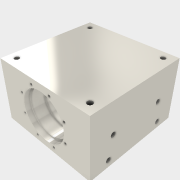
# Autodesk Inventor part: PWTR-0045
Saved by Autodesk Inventor 2021.1 (Build 251245000, 245)
## iProperties
Created: 2020-08-27
Part Number: PWTR-0045
Material: Aluminum 6061
Document SubType Name: Modeling
Designer: alid
Density: 2.7 g/cm^3
Appearance: Titanium - Polished
Description: Transfer Box Casing
Mass: 2475.75 g
Surface Area: 1069.23 cm^2
Volume: 916.945 cm^3
Author: alid
Revision Number: A
Autodesk Inventor part; units mm, degrees
ref_plane "YZ Plane" through (0, 0, 0) normal (1, 0, 0) x (0, 1, 0)
ref_plane "XZ Plane" through (0, 0, 0) normal (0, 1, 0) x (-1, 0, 0)
ref_plane "XY Plane" through (0, 0, 0) normal (0, 0, 1) x (1, 0, 0)
sketch "Sketch1" plane through (0, 0, 0) normal (0, 0, 1) x (1, 0, 0)
  line L0 (-65, -65) -> (65, -65)
  line L1 (65, -65) -> (65, 65)
  line L2 (65, 65) -> (-65, 65)
  line L3 (-65, 65) -> (-65, -65)
  line L4 (-65, -65) -> (65, 65) construction
  line L5 (65, -65) -> (-65, 65) construction
  circle A0 centre (0, 0) radius 50 construction
  circle A1 centre (0, 0) radius 75 construction
  point P0 (35.3553, 35.3553)
  point P1 (53.033, 53.033)
  dimension "d4" = 100
  dimension "d22" = 150
  dimension "d0" = 130
  dimension "d1" = 130
  constraints: 12 end point, 2 coincident, 2 midpoint, 2 parallel, 2 point on line, 1 horizontal, 1 perpendicular, 6 other
  measures "d0" distance of L2.end L1.end
  measures "d1" distance of L1.end L0.end
extrude "Extrusion1" add sketch "Sketch1" along normal blind 80
hole "Hole1" at (35.3553, 35.3553, 0) direction (0, 0, 1) diameter 6.647 depth 22.2 tip angle 118 thread size "M8x1.25" class "6H" standard "ISO Metric profile"
hole "Hole2" at (0, 0, 0) direction (0, 0, 1) diameter 75 depth 70
pattern_circular "Circular Pattern1" count 4 over 360 about axis through (0, 0, -10) along (0, 0, 1) of "Hole1"
hole "Hole3" at (53.033, 53.033, 0) direction (0, 0, 1) diameter 6.647 end through all thread size "M8x1.25" class "6H" standard "ISO Metric profile"
pattern_circular "Circular Pattern2" count 4 over 360 about axis through (0, 0, -10) along (0, 0, 1) of "Hole3"
sketch "Sketch2" plane through (0, 0, 0) normal (0, 1, 0) x (-1, 0, 0)
  line L0 (0, 40) -> (65, 40)
  line L1 (0, 66) -> (0, 40)
  line L2 (65, 47.2135) -> (65, 40)
  line L3 (65, 0) -> (65, 80) projected
  line L4 (0, 66) -> (41, 66)
  line L5 (41, 66) -> (41, 69)
  line L6 (41, 69) -> (65, 69)
  line L7 (0, 61) -> (-49.5, 61)
  line L8 (-49.5, 61) -> (-52.5, 58)
  line L9 (-52.5, 58) -> (-52.5, 50)
  line L10 (-52.5, 50) -> (-65, 50)
  line L11 (-65, 50) -> (-65, 40)
  line L12 (-65, 40) -> (0, 40)
  line L13 (58, 69) -> (58, 71)
  line L14 (58, 71) -> (65, 71)
  line L15 (65, 69) -> (65, 71)
  point P0 (0, 0)
  dimension "d36" = 40
  dimension "d42" = 41
  dimension "d43" = 26
  dimension "d44" = 29
  dimension "d45" = 42
  dimension "d46" = 135
  dimension "d47" = 3
  dimension "d48" = 20
  dimension "d50" = 65
  dimension "d51" = 49.5
  dimension "d59" = 7
  dimension "d60" = 31
  constraints: 30 end point, 8 perpendicular, 5 point on line, 2 horizontal, 2 vertical, 2 vertical alignment, 1 midpoint, 1 parallel
  measures "d36" distance from line of L3.start L0
  measures "d42" distance between parallel lines of L5 L1
  measures "d43" distance from line of L0.start L4
  measures "d44" distance from line of L0.start L6
  measures "d45" diameter of L7 L12
  measures "d46" angle of L9 L8
  measures "d47" horizontal distance of L7.end L8.end
  measures "d48" diameter of L10 L12
  measures "d50" distance from line of L0.start L11
  measures "d51" distance from line of L7.end L1
  measures "d59" distance of L13.end L14.end
  measures "d60" distance from line of L0.start L14
revolve "Revolution1" cut sketch "Sketch2" angle 360 about axis through (0, 0, 40) along (-1, 0, 0)
sketch "Sketch3" plane through (65, -65, 0) normal (1, 0, 0) x (0, 0, -1)
  circle A0 centre (-40, 65) radius 10 projected
  point P0 (0, 65)
  constraints: 1 coincident
hole "Hole4" at (65, 0, 40) direction (-1, 0, 0) diameter 30 depth 7
sketch "Sketch4" plane through (-65, -65, 0) normal (-1, 0, 0) x (0, 0, 1)
  circle A0 centre (40, 65) radius 31 projected
  circle A1 centre (40, 65) radius 40 construction
  circle A2 centre (40, 65) radius 35 construction
  line L0 (40, 65) -> (75, 65) construction
  line L1 (40, 65) -> (72.3358, 51.6061) construction
  point P0 (0, 65)
  dimension "d61" = 80
  dimension "d62" = 70
  dimension "d63" = 22.5
  constraints: 4 end point, 2 centre point, 2 coincident, 2 point on circle, 1 horizontal
  measures "d61" diameter of A1
  measures "d62" diameter of A2
  measures "d63" angle of L1 L0
hole "Hole5" at (-65, -13.3939, 72.3358) direction (1, 0, 0) diameter 3.242 depth 11.8 thread size "M4x0.7" class "6H" standard "ISO Metric profile"
pattern_circular "Circular Pattern3" count 8 over 360 about axis through (-61.5, 0, 40) along (1, 0, 0) of "Hole5"
sketch "Sketch5" plane through (-65, -65, 0) normal (0, -1, 0) x (1, 0, 0)
  line L0 (25, 0) -> (105, 0)
  line L1 (100, 50) -> (30, 50)
  line L2 (109.8639, 41.644) -> (114.8639, 11.644)
  circle A0 centre (30, 40) radius 10
  circle A1 centre (25, 10) radius 10
  circle A2 centre (100, 40) radius 10
  circle A3 centre (105, 10) radius 10
  line L3 (20.1361, 41.644) -> (15.1361, 11.644)
  line L4 (0, 0) -> (130, 0) projected
  point P0 (65, 0)
  point P1 (-44.8639, 16.644)
  point P2 (65, 50)
  point P3 (65, 0)
  dimension "d74" = 70
  dimension "d75" = 50
  dimension "d77" = 80
  dimension "d78" = 20
  constraints: 8 end point, 8 point on circle, 8 tangent, 4 centre point, 3 coincident, 3 equal radius, 3 midpoint, 1 horizontal, 1 parallel, 1 vertical alignment
  measures "d74" distance of L1.start L1.end
  measures "d75" distance between parallel lines of L0 L1
  measures "d77" distance of L0.start L0.end
  measures "d78" diameter of A0
hole "Hole6" at (35, -65, 40) direction (0, 1, 0) diameter 6.647 depth 22.2 tip angle 118 thread size "M8x1.25" class "6H" standard "ISO Metric profile"
pattern_sketch "Sketch Driven Pattern1" of "Hole6" from (35, -65, 40) copies at (40, -65, 10) at (-40, -65, 10) at (-35, -65, 40)
equation "\"d1\" = d0"
body "Solid1"
body "Solid2"
body "Solid3"
